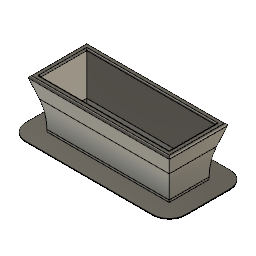
smmb_coin-thrower-top (Autodesk Fusion 360 design; units mm, degrees)
Autodesk Fusion 360 part; units mm, degrees
sketch "Sketch1" plane through (0, 0, 0) normal (0, 0, 1) x (1, 0, 0)
  line L0 (0, 0) -> (28.5, 0)
  line L1 (28.5, 0) -> (28.5, 3.5)
  line L2 (28.5, 3.5) -> (0, 3.5)
  line L3 (0, 3.5) -> (0, 0)
  line L4 (-2, -2) -> (30.5, -2)
  line L5 (30.5, -2) -> (30.5, 5.5)
  line L6 (30.5, 5.5) -> (-2, 5.5)
  line L7 (-2, 5.5) -> (-2, -2)
  line L8 (-2.3, -2.3) -> (30.8, -2.3)
  line L9 (30.8, -2.3) -> (30.8, 5.8)
  line L10 (30.8, 5.8) -> (-2.3, 5.8)
  line L11 (-2.3, 5.8) -> (-2.3, -2.3)
  line L12 (-4.3, -4.3) -> (32.8, -4.3)
  line L13 (32.8, -4.3) -> (32.8, 7.8)
  line L14 (32.8, 7.8) -> (-4.3, 7.8)
  line L15 (-4.3, 7.8) -> (-4.3, -4.3)
  line L16 (38.5, 13.5) -> (-10, 13.5)
  line L17 (-10, 13.5) -> (-10, -10)
  line L18 (-10, -10) -> (38.5, -10)
  line L19 (38.5, -10) -> (38.5, 13.5)
  dimension "d1" = 28.5
  dimension "d2" = 3.5
  dimension "d3" = 2
  dimension "d6" = 2.3
  dimension "d7" = 4.3
  dimension "d22" = 10
  constraint horizontal L0
  constraint vertical L1
  constraint horizontal L2
  constraint vertical L3
  constraint coincident L0.start L3.end
  measures "d1" distance of L0.start L0.end
  measures "d2" distance of L0.start L2.end
extrude "Extrude2" add sketch "Sketch1" along normal blind 5 contours L12 L13 L14 L15
sketch "Sketch2" plane through (-2.3, 0, 0) normal (1, 0, 0) x (0, 1, 0)
  line L0 (-2.3, 0) -> (5.8, 0)
  line L1 (5.8, 0) -> (5.8, 5)
  line L2 (5.8, 5) -> (-2.3, 5)
  line L3 (-2.3, 5) -> (-2.3, 0)
  circle A0 centre (1.75, 2.5) radius 1.25
  line L4 (-4.3, 0) -> (7.8, 0)
  line L5 (7.8, 0) -> (7.8, 5)
  line L6 (7.8, 5) -> (-4.3, 5)
  line L7 (-4.3, 5) -> (-4.3, 0)
  line L8 (1.75, 3.75) -> (1.75, 1.25)
  circle A1 centre (1.75, 2.5) radius 1.1
  dimension "d10" = 2.5
  dimension "d11" = 6.05
  dimension "d12" = 2.5
  dimension "d13" = 2.2
  constraint coincident A0 L8.start
  constraint coincident A0 L8.end
  constraint vertical L8
  constraint concentric A0 A1
  measures "d10" distance of L2 A0.centre
  measures "d11" distance of A0.centre L7
  measures "d12" diameter of A0
  measures "d13" diameter of A1
sketch "Sketch3" plane through (30.8, 0, 0) normal (-1, 0, 0) x (0, -1, 0)
  line L0 (-5.8, 0) -> (2.3, 0)
  line L1 (2.3, 0) -> (2.3, 5)
  line L2 (2.3, 5) -> (-5.8, 5)
  line L3 (-5.8, 5) -> (-5.8, 0)
  circle A0 centre (-1.75, 2.5) radius 1.1
  line L4 (-1.75, 3.75) -> (-1.75, 1.25)
revolve "Revolve1" add sketch "Sketch2" angle 360 about axis through (-2.3, 1.75, 3.75) along (0, 0, -1) contours L8 A1 picked at (1.4633, 2.2714)
revolve "Revolve2" add sketch "Sketch3" angle 360 about axis through (30.8, 1.75, 3.75) along (0, 0, -1) contours A0 L4 picked at (-2.1156, 2.5274)
ref_plane "WorkPlane1" through (14.25, 1.75, 15) normal (0, 0, 1) x (1, 0, 0)
sketch "Sketch4" plane through (14.25, 1.75, 15) normal (0, 0, 1) x (1, 0, 0)
  line L0 (-16.55, -4.05) -> (-16.55, 4.05)
  line L1 (-16.55, 4.05) -> (16.55, 4.05)
  line L2 (16.55, 4.05) -> (16.55, -4.05)
  line L3 (16.55, -4.05) -> (-16.55, -4.05)
  line L4 (-18.55, 6.05) -> (-18.55, -6.05)
  line L5 (-18.55, -6.05) -> (18.55, -6.05)
  line L6 (18.55, -6.05) -> (18.55, 6.05)
  line L7 (18.55, 6.05) -> (-18.55, 6.05)
  line L8 (-21.55, -9.05) -> (21.55, -9.05)
  line L9 (21.55, -9.05) -> (21.55, 9.05)
  line L10 (21.55, 9.05) -> (-21.55, 9.05)
  line L11 (-21.55, 9.05) -> (-21.55, -9.05)
  line L12 (-19.55, -7.05) -> (19.55, -7.05)
  line L13 (19.55, -7.05) -> (19.55, 7.05)
  line L14 (19.55, 7.05) -> (-19.55, 7.05)
  line L15 (-19.55, 7.05) -> (-19.55, -7.05)
  dimension "d17" = 3
  dimension "d18" = 1
sketch "Sketch5" plane through (0, 0, 5) normal (0, 0, 1) x (-1, 0, 0)
  line L0 (2.3, 2.3) -> (2.3, -5.8)
  line L1 (2.3, -5.8) -> (-30.8, -5.8)
  line L2 (-30.8, -5.8) -> (-30.8, 2.3)
  line L3 (-30.8, 2.3) -> (2.3, 2.3)
  line L4 (4.3, -7.8) -> (4.3, 4.3)
  line L5 (4.3, 4.3) -> (-32.8, 4.3)
  line L6 (-32.8, 4.3) -> (-32.8, -7.8)
  line L7 (-32.8, -7.8) -> (4.3, -7.8)
loft "Loft1" add profiles "Sketch5", "Sketch4" section 1 section 2 contours L8 L9 L10 L11
loft "Loft2" cut profiles "Sketch4", "Sketch5" section 1 contours L0 L1 L2 L3 | L4 L5 L6 L7 | L12 L13 L14 L15 section 2 contours L0 L1 L2 L3
fillet "Fillet1" radius 0.5 4 edges at (-7.3, 1.75, 15) (14.25, 10.8, 15) (14.25, -7.3, 15) (35.8, 1.75, 15)
fillet "Fillet1" radius 0.5 4 edges at (14.25, 8.8, 15) (33.8, 1.75, 15) (14.25, -5.3, 15) (-5.3, 1.75, 15)
fillet "Fillet2" radius 28 4 edges at (14.25, -4.3, 5) (-4.3, 1.75, 5) (14.25, 7.8, 5) (32.8, 1.75, 5)
extrude "Extrude3" add sketch "Sketch1" along normal blind 0.25 contours L16 L17 L18 L19
fillet "Fillet3" radius 5 4 edges at (38.5, -10, 0.125) (38.5, 13.5, 0.125) (-10, -10, 0.125) (-10, 13.5, 0.125)
